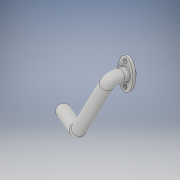
# Autodesk Inventor part: Component 51(Intake Pipe)
Saved by Autodesk Inventor 2018 (Build 220112000, 112)
## iProperties
Created: 2023-04-11
Part Number: Component 51(Intake Pipe)
Material: Generic
Document SubType Name: Modeling
Designer: Habib Mohamed
Density: 1 g/cm^3
Appearance: Default
Author: Habib Mohamed
Autodesk Inventor part; units mm, degrees
ref_plane "YZ Plane" through (0, 0, 0) normal (1, 0, 0) x (0, 1, 0)
ref_plane "XY Plane" through (0, 0, 0) normal (0, 0, 1) x (1, 0, 0)
sketch "Sketch1" plane through (0, 0, 0) normal (0, 0, 1) x (1, 0, 0)
  line L0 (0, 0) -> (0, 10) construction
  line L1 (0, 0) -> (6, 0) construction
  circle A0 centre (0, 0) radius 3.5
  circle A1 centre (0, 7) radius 1.5
  circle A2 centre (0, -7) radius 1.5
  ellipse E0 centre (0, 0) end of major axis (6, 0) minor radius 10
  dimension "d0" = 10
  dimension "d1" = 6
  dimension "d2" = 7
  dimension "d4" = 3
  dimension "d5" = 3
  dimension "d6" = 7
  dimension "d7" = 7
  constraints: 4 end point, 3 centre point, 2 coincident, 2 horizontal, 1 point on line, 1 vertical, 1 vertical alignment, 4 other
  measures "d0" distance of L0.start L0.end
  measures "d1" distance of L0.start L1.end
  measures "d2" diameter of A0
  measures "d4" diameter of A1
  measures "d5" diameter of A2
  measures "d6" distance from line of L1 A1.centre
  measures "d7" distance from line of A2.centre L1
extrude "Extrusion1" add sketch "Sketch1" along normal blind 2
sketch "Sketch2" plane through (0, 0, 0) normal (1, 0, 0) x (0, 1, 0)
  line L0 (0, -2) -> (0, 5) construction
  point P0 (0, 0)
  dimension "d10" = 2
  dimension "d11" = 7
  constraints: 2 end point, 1 vertical
  measures "d10" distance of L0.start point (0, 0)
  measures "d11" distance of L0.start L0.end
ref_plane "Work Plane1" through (0, -45, 0) normal (0, 1, 0) x (-1, 0, 0)
sketch "Sketch3" plane through (0, -45, 0) normal (0, 1, 0) x (-1, 0, 0)
  line L0 (0, 0) -> (0, -83.2566) construction
  line L1 (69.478, -15.021) -> (43.1392, -69.7245) construction
  line L2 (69.478, -15.021) -> (42.448, -2.0065) construction
  dimension "d13" = 25.71
  dimension "d14" = 69.478
  dimension "d16" = 15.021
  dimension "d17" = 30
  dimension "d18" = 90
  constraints: 6 end point, 1 vertical
  measures "d13" angle of L1 L0
  measures "d14" distance from line of L0 L1.start
  measures "d16" vertical distance of L1.start L0.start
  measures "d17" distance of L1.start L2.end
  measures "d18" angle of L2 L1
ref_plane "Work Plane2" through (-69.478, -45, -15.021) normal (0.9010013, 0, 0.4338163) x (0, 1, 0)
sketch "Sketch4" plane through (-69.478, -45, -15.021) normal (0.9010013, 0, 0.4338163) x (0, 1, 0)
  circle A0 centre (0, 0) radius 4
  circle A1 centre (0, 0) radius 3.5
  point P0 (45, -16.6068)
  dimension "d19" = 8
  dimension "d20" = 7
  constraints: 2 centre point, 1 coincident
  measures "d19" diameter of A0
  measures "d20" diameter of A1
sketch3d "3D Sketch1"
  line L0 (-69.478, -45, -15.021) -> (-44.345, -45, -2.9199)
  arc A0 (-44.345, -45, -2.9199) -> (-41.0389, -43.5063, -1.5416) centre (-44.0679, -40.0409, -3.4952) ccw
  line L1 (-41.0389, -43.5063, -1.5416) -> (-4.1885, -4.4404, 10.6179)
  arc A1 (-4.1885, -4.4404, 10.6179) -> (0, 0, 5.7414) centre (-3.4309, -3.6372, 5.7414) ccw
  line L2 (0, 0, 5.7414) -> (0, 0, 5)
  line L3 (0, 0, 5) -> (0, 0, -2)
  dimension "d21" = 5
  dimension "d22" = 5
  dimension "d23" = 7
sweep "Sweep1" add profiles "Sketch4" path "3D Sketch1"
fillet "Fillet1" radius 0.5 1 edges at (3.5625, -1.819, 2)
equation "\"d7\" = d6"
equation "\"d22\" = d21"
body "Solid1"
